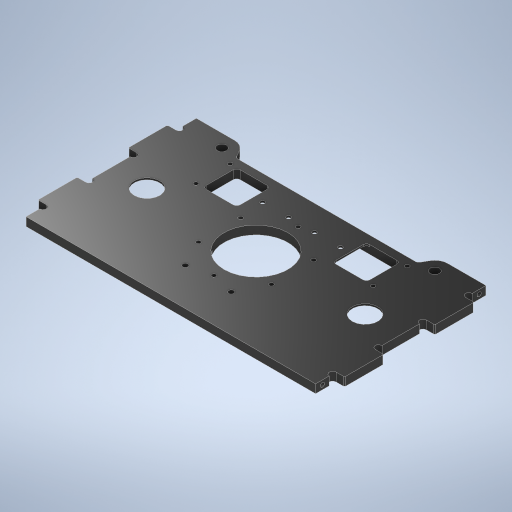
# Autodesk Inventor part: TorsoUpperFrame
Saved by Autodesk Inventor 2024.2 (Build 282272000, 272)
## iProperties
Created: 2024-01-05
Part Number: TorsoUpperFrame
Material: Aluminum 7075
Document SubType Name: Modeling
Designer: Masato Kubotera
Density: 2.81 g/cm^3
Appearance: Glossy - Black
Vendor: meviy
Mass: 108.003 g
Surface Area: 393.241 cm^2
Volume: 38.4352 cm^3
Author: Masato Kubotera
Autodesk Inventor part; units mm, degrees
ref_plane "YZ Plane" through (0, 0, 0) normal (1, 0, 0) x (0, 1, 0)
ref_plane "XZ Plane" through (0, 0, 0) normal (0, 1, 0) x (-1, 0, 0)
ref_plane "XY Plane" through (0, 0, 0) normal (0, 0, 1) x (1, 0, 0)
sketch "Sketch1" plane through (0, 0, 0) normal (0, 0, 1) x (1, 0, 0)
  line L0 (-50, -90) -> (50, -90)
  line L1 (50, -90) -> (50, 90)
  line L2 (50, 90) -> (-50, 90)
  line L3 (-50, 90) -> (-50, -90)
  line L4 (-50, -90) -> (50, 90) construction
  line L5 (50, -90) -> (-50, 90) construction
  line L6 (-50, 0) -> (50, 0)
  line L7 (0, -90) -> (0, 90) construction
  circle A0 centre (0, 0) radius 18.75
  line L8 (-12, -16) -> (31, -16) construction
  line L9 (31, -16) -> (31, 16) construction
  line L10 (31, 16) -> (-12, 16) construction
  line L11 (-12, 16) -> (-12, -16) construction
  line L12 (-12, -16) -> (31, 16) construction
  line L13 (31, -16) -> (-12, 16) construction
  line L14 (1, -13.5) -> (28, -13.5) construction
  line L15 (28, -13.5) -> (28, 13.5) construction
  line L16 (28, 13.5) -> (1, 13.5) construction
  line L17 (1, 13.5) -> (1, -13.5) construction
  line L18 (1, -13.5) -> (28, 13.5) construction
  line L19 (28, -13.5) -> (1, 13.5) construction
  line L20 (9.61, -16.1) -> (31.1, -16.1)
  line L21 (31.1, -16.1) -> (31.1, 16.1)
  line L22 (31.1, 16.1) -> (9.61, 16.1)
  line L23 (50, 85) -> (38, 85)
  line L24 (38, 85) -> (38, 90)
  line L25 (-15, 90) -> (-15, 85)
  line L26 (-15, 85) -> (15, 85)
  line L27 (15, 85) -> (15, 90)
  arc A1 (38, 85) -> (42, 85) centre (40, 85) ccw
  arc A2 (11, 85) -> (15, 85) centre (13, 85) ccw
  line L28 (-50, 85) -> (-38, 85)
  line L29 (-38, 85) -> (-38, 90)
  arc A3 (-42, 85) -> (-38, 85) centre (-40, 85) ccw
  arc A4 (-15, 85) -> (-11, 85) centre (-13, 85) ccw
  line L30 (46, 85) -> (46, 79) construction
  line L31 (-46, 85) -> (-46, 79) construction
  circle A5 centre (0, 0) radius 29 construction
  line L32 (-41.5, 0) -> (-41.5, 53.2624)
  line L33 (-41.5, 53.2624) -> (-50, 58.1699)
  circle A6 centre (-42.5, 62.5) radius 7.5 construction
  circle A7 centre (-42.5, 62.5) radius 5 construction
  line L34 (-70, -90.6743) -> (-70, 90) construction
  line L35 (70, -90.6743) -> (70, 90) construction
  line L36 (-50, 62.5) -> (-37.5, 62.5) construction
  circle A8 centre (-42.5, -62.5) radius 7.5 construction
  circle A9 centre (-42.5, -62.5) radius 5 construction
  line L37 (50, -85) -> (38, -85)
  line L38 (38, -85) -> (38, -90)
  line L39 (-15, -90) -> (-15, -85)
  line L40 (-15, -85) -> (15, -85)
  line L41 (15, -85) -> (15, -90)
  arc A10 (42, -85) -> (38, -85) centre (40, -85) ccw
  arc A11 (15, -85) -> (11, -85) centre (13, -85) ccw
  arc A12 (-11, -85) -> (-15, -85) centre (-13, -85) ccw
  line L42 (-38, -85) -> (-38, -90)
  arc A13 (-38, -85) -> (-42, -85) centre (-40, -85) ccw
  line L43 (-50, -85) -> (-38, -85)
  line L44 (-41.5, 0) -> (-41.5, -53.2624)
  line L45 (-41.5, -53.2624) -> (-50, -58.1699)
  line L46 (-35.6, 29.25) -> (-17.9, 29.25) construction
  line L47 (-17.4, 28.75) -> (-36.1, 28.75) construction
  line L48 (-36.6858, 30.1642) -> (-36.6858, 46.0358)
  line L49 (-35.6, 46.95) -> (-35.6, 29.25) construction
  line L50 (-35.6, 46.95) -> (-17.9, 29.25) construction
  line L51 (-17.9, 46.95) -> (-35.6, 29.25) construction
  line L52 (-36.1, 47.45) -> (-17.4, 47.45) construction
  line L53 (-36.1, 47.45) -> (-17.4, 28.75) construction
  line L54 (-17.4, 47.45) -> (-36.1, 28.75) construction
  line L55 (-36.6858, 48.0358) -> (-16.8142, 28.1642) construction
  line L56 (-16.8142, 48.0358) -> (-36.6858, 28.1642) construction
  arc A14 (-34.6858, 48.0358) -> (-36.6858, 46.0358) centre (-34.6858, 46.0358) ccw
  line L57 (-16.8142, 46.0358) -> (-16.8142, 30.1642)
  line L58 (-17.9, 29.25) -> (-17.9, 46.95) construction
  line L59 (-17.4, 47.45) -> (-17.4, 28.75) construction
  line L60 (-18.8142, 28.1642) -> (-34.6858, 28.1642)
  arc A15 (-36.6858, 30.1642) -> (-34.6858, 28.1642) centre (-34.6858, 30.1642) ccw
  arc A16 (-18.8142, 28.1642) -> (-16.8142, 30.1642) centre (-18.8142, 30.1642) ccw
  line L61 (-34.6858, 48.0358) -> (-18.8142, 48.0358)
  arc A17 (-16.8142, 46.0358) -> (-18.8142, 48.0358) centre (-18.8142, 46.0358) ccw
  line L62 (-17.9, 46.95) -> (-35.6, 46.95) construction
  line L63 (-36.1, 28.75) -> (-36.1, 47.45) construction
  line L64 (-36.6858, -30.1642) -> (-36.6858, -46.0358)
  line L65 (-34.6858, -48.0358) -> (-18.8142, -48.0358)
  line L66 (-35.6, -46.95) -> (-35.6, -29.25) construction
  line L67 (-17.9, -46.95) -> (-35.6, -46.95) construction
  line L68 (-36.1, -28.75) -> (-36.1, -47.45) construction
  line L69 (-36.1, -47.45) -> (-17.4, -47.45) construction
  line L70 (-35.6, -29.25) -> (-17.9, -29.25) construction
  line L71 (-35.6, -46.95) -> (-17.9, -29.25) construction
  line L72 (-17.9, -46.95) -> (-35.6, -29.25) construction
  line L73 (-18.8142, -28.1642) -> (-34.6858, -28.1642)
  line L74 (-16.8142, -48.0358) -> (-36.6858, -28.1642) construction
  line L75 (-36.6858, -48.0358) -> (-16.8142, -28.1642) construction
  line L76 (-17.4, -28.75) -> (-36.1, -28.75) construction
  line L77 (-36.1, -47.45) -> (-17.4, -28.75) construction
  line L78 (-17.4, -47.45) -> (-36.1, -28.75) construction
  line L79 (-17.9, -29.25) -> (-17.9, -46.95) construction
  line L80 (-17.4, -47.45) -> (-17.4, -28.75) construction
  arc A18 (-16.8142, -30.1642) -> (-18.8142, -28.1642) centre (-18.8142, -30.1642) ccw
  line L81 (-16.8142, -46.0358) -> (-16.8142, -30.1642)
  arc A19 (-34.6858, -28.1642) -> (-36.6858, -30.1642) centre (-34.6858, -30.1642) ccw
  arc A20 (-18.8142, -48.0358) -> (-16.8142, -46.0358) centre (-18.8142, -46.0358) ccw
  arc A21 (-36.6858, -46.0358) -> (-34.6858, -48.0358) centre (-34.6858, -46.0358) ccw
  arc A22 (0, 16) -> (-12, 10.583) centre (0, 0) ccw construction
  arc A23 (-12, -10.583) -> (0, -16) centre (0, 0) ccw construction
  line L82 (-26.75, 38.1) -> (-26.75, -38.1) construction
  line L83 (-14.5, 55) -> (-27.6628, 55)
  arc A24 (-39.3295, 80) -> (-41.0778, 77.0287) centre (-39.3295, 78) ccw
  line L84 (-41.5, 16) -> (-37.5, 16) construction
  line L85 (-41.5, -16) -> (-37.5, -16) construction
  line L86 (-37.25, -49) -> (-16.25, -49) construction
  line L87 (-14.25, -47) -> (-14.25, 47) construction
  line L88 (-16.25, 49) -> (-37.25, 49) construction
  line L89 (-39.25, 47) -> (-39.25, -47) construction
  line L90 (-39.25, -49) -> (-14.25, 49) construction
  line L91 (-14.25, -49) -> (-39.25, 49) construction
  line L92 (-16.75, 52) -> (-36.75, 52) construction
  circle A25 centre (-16.75, 52) radius 1 construction
  circle A26 centre (-16.75, 52) radius 2 construction
  line L93 (-39, -55) -> (-14.5, -55) construction
  line L94 (-12.5, -53) -> (-12.5, 53) construction
  line L95 (-14.5, 55) -> (-39, 55) construction
  line L96 (-41, 53) -> (-41, -53) construction
  line L97 (-41, -55) -> (-12.5, 55) construction
  line L98 (-12.5, -55) -> (-41, 55) construction
  arc A27 (-12.5, 53) -> (-14.5, 55) centre (-14.5, 53) ccw
  arc A28 (-39, 55) -> (-41, 53) centre (-39, 53) ccw construction
  arc A29 (-41, -53) -> (-39, -55) centre (-39, -53) ccw construction
  arc A30 (-14.5, -55) -> (-12.5, -53) centre (-14.5, -53) ccw construction
  arc A31 (-37.25, 49) -> (-39.25, 47) centre (-37.25, 47) ccw construction
  arc A32 (-14.25, 47) -> (-16.25, 49) centre (-16.25, 47) ccw construction
  arc A33 (-16.25, -49) -> (-14.25, -47) centre (-16.25, -47) ccw construction
  arc A34 (-39.25, -47) -> (-37.25, -49) centre (-37.25, -47) ccw construction
  line L99 (-17.75, 22.5) -> (-35.75, 22.5) construction
  line L100 (-35.75, 22.5) -> (-35.75, -22.5) construction
  line L101 (-35.75, -22.5) -> (-17.75, -22.5) construction
  line L102 (-17.75, -22.5) -> (-17.75, 22.5) construction
  line L103 (-17.75, 22.5) -> (-35.75, -22.5) construction
  line L104 (-35.75, 22.5) -> (-17.75, -22.5) construction
  line L105 (41.0778, 77.0287) -> (13.0754, 26.6244)
  line L106 (15.6978, 25.1674) -> (43.2517, 74.7643)
  line L107 (47, 73.7931) -> (47, 3.5)
  line L108 (29.1, 18.1) -> (17.9933, 18.1)
  arc A35 (47, 73.7931) -> (43.2517, 74.7643) centre (45, 73.7931) ccw
  arc A36 (16.0474, 20.5621) -> (17.9933, 18.1) centre (17.9933, 20.1) ccw
  line L109 (-36.6858, 23.1642) -> (-36.6858, 0)
  line L110 (-34.37, -22.5) -> (-34.37, 22.5) construction
  line L111 (-29.25, 5.12) -> (-24.25, 5.12) construction
  line L112 (-24.25, 5.12) -> (-24.25, 10.12) construction
  line L113 (-24.25, 10.12) -> (-29.25, 10.12) construction
  line L114 (-29.25, 10.12) -> (-29.25, 5.12) construction
  line L115 (-29.25, 5.12) -> (-24.25, 10.12) construction
  line L116 (-24.25, 5.12) -> (-29.25, 10.12) construction
  circle A37 centre (-26.75, 7.62) radius 1.5 construction
  line L117 (-32.99, -22.5) -> (-32.99, 22.5) construction
  line L118 (-29.25, 25.36) -> (-29.25, 20.36) construction
  line L119 (-29.25, 20.36) -> (-24.25, 20.36) construction
  line L120 (-24.25, 20.36) -> (-24.25, 25.36) construction
  circle A38 centre (-26.75, 22.86) radius 1.5 construction
  line L121 (-24.25, 25.36) -> (-29.25, 25.36) construction
  arc A39 (-23.5471, 4.0762) -> (-29, 0) centre (-24.75, 0) ccw
  arc A40 (-23.5471, 4.0762) -> (-21.0458, 5.4896) centre (-22.9811, 5.9944) ccw
  arc A41 (-17.2299, 13.2738) -> (-21.0458, 5.4896) centre (0, 0) ccw
  arc A42 (5.7687, 20.971) -> (-5.7687, 20.971) centre (0, 0) ccw
  arc A43 (5.7687, 20.971) -> (8.2434, 22.4305) centre (6.2992, 22.8994) ccw
  arc A44 (11.6624, 25.624) -> (13.0754, 26.6244) centre (11.3271, 27.5956) ccw
  arc A45 (15.6978, 25.1674) -> (15.4533, 24.3645) centre (17.4462, 24.1961) ccw
  line L122 (-12.5, 27.3962) -> (-12.5, 53)
  arc A46 (11.6624, 25.624) -> (8.2434, 22.4305) centre (12.375, 21.4341) ccw
  arc A47 (-8.2434, 22.4305) -> (-5.7687, 20.971) centre (-6.2992, 22.8994) ccw
  arc A48 (-8.2434, 22.4305) -> (-11.1, 25.4884) centre (-12.375, 21.4341) ccw
  arc A49 (-12.5, 27.3962) -> (-11.1, 25.4884) centre (-10.5, 27.3962) ccw
  line L123 (-39.3295, 80) -> (39.3295, 80)
  arc A50 (41.0778, 77.0287) -> (39.3295, 80) centre (39.3295, 78) ccw
  line L124 (45, 1.5) -> (35.1, 1.5)
  line L125 (33.1, 3.5) -> (33.1, 14.1)
  arc A51 (45, 1.5) -> (47, 3.5) centre (45, 3.5) ccw
  arc A52 (33.1, 3.5) -> (35.1, 1.5) centre (35.1, 3.5) ccw
  arc A53 (33.1, 14.1) -> (29.1, 18.1) centre (29.1, 14.1) ccw
  line L126 (-41.0778, 77.0287) -> (-29.4111, 56.0287)
  arc A54 (15.6978, 25.1674) -> (15.6898, 23.2395) centre (17.4462, 24.1961) ccw
  arc A55 (16.0474, 20.5621) -> (15.6898, 23.2395) centre (12.375, 21.4341) ccw
  arc A56 (-29.4111, 56.0287) -> (-27.6628, 55) centre (-27.6628, 57) ccw
  line L127 (-36.6858, 23.1642) -> (-36.6858, 30.1642)
  line L128 (-16.8142, 30.1642) -> (-16.8142, 14.4944)
  arc A57 (-17.2299, 13.2738) -> (-16.8142, 14.4944) centre (-18.8142, 14.4944) ccw
  circle A58 centre (0, 64) radius 7.5
  point P0 (9.5, 0)
  point P1 (14.5, 0)
  point P2 (24.75, 0)
  point P3 (-12.375, 21.4341)
  point P4 (-12.375, -21.4341)
  point P5 (12.375, -21.4341)
  point P6 (-37.5, -62.5)
  point P7 (46, -85)
  point P8 (-46, -85)
  point P9 (-50, -58.1699)
  point P10 (-50, -85)
  point P11 (-38, -90)
  point P12 (-11, -85)
  point P13 (38, -90)
  point P14 (50, -85)
  point P15 (-11, 85)
  point P16 (-50, 85)
  point P17 (50, 69.4499)
  point P18 (50, 77.5499)
  point P19 (-46, -79)
  point P20 (-26.75, 38.1)
  point P21 (-26.75, 38.1)
  point P22 (-26.75, -38.1)
  point P23 (-26.75, 38.1)
  point P24 (18.75, 0)
  point P25 (-18.75, 0)
  point P26 (-35, 55)
  point P27 (-28.8396, 55)
  point P28 (-26.75, 0)
  point P29 (-16.75, -52)
  point P30 (-36.75, -52)
  point P31 (43.8396, 82)
  point P32 (42.2091, 72.8876)
  point P33 (47, 72.8875)
  point P34 (47, 1.5)
  point P35 (33.1, 18.1)
  point P36 (-12.5, 51.9999)
  point P37 (40, 83)
  point P38 (-16.8142, 24.516)
  point P39 (-16.8142, 13.7965)
  dimension "d24" = 58
  dimension "d26" = 10
  dimension "d0" = 100
  dimension "d1" = 180
  dimension "d2" = 37.5
  dimension "d3" = 43
  dimension "d4" = 32
  dimension "d5" = 27
  dimension "d6" = 27
  dimension "d7" = 9.5
  dimension "d8" = 8.5
  dimension "d9" = 0.1
  dimension "d10" = 0.1
  dimension "d15" = 360
  dimension "d17" = 49.5
  dimension "d18" = 5
  dimension "d19" = 30
  dimension "d20" = 12
  dimension "d21" = 2
  dimension "d22" = 6
  dimension "d23" = 8
  dimension "d25" = 15
  dimension "d27" = 140
  dimension "d29" = 125
  dimension "d77" = 2
  dimension "d78" = 17.7
  dimension "d79" = 17.7
  dimension "d80" = 0.5
  dimension "d81" = 76.2
  dimension "d100" = 4
  dimension "d101" = 32
  dimension "d128" = 8.5
  dimension "d130" = 29.5
  dimension "d131" = 25
  dimension "d132" = 98
  dimension "d133" = 2
  dimension "d134" = 4
  dimension "d135" = 20
  dimension "d138" = 0.5
  dimension "d139" = 6
  dimension "d140" = 2
  dimension "d141" = 2
  dimension "d149" = 18
  dimension "d150" = 45
  dimension "d151" = 2
  dimension "d153" = 3
  dimension "d157" = 3
  dimension "d173" = 15.24
  dimension "d176" = 5
  dimension "d178" = 3
  dimension "d181" = 15.24
  dimension "d184" = 15.24
  dimension "d191" = 3
  dimension "d205" = 5
  dimension "d212" = 2
  dimension "d213" = 3
  dimension "d215" = 4
  dimension "d216" = 3
  dimension "d218" = 60
  dimension "d223" = 2
  dimension "d225" = 15
  dimension "d226" = 21
  constraints: 258 end point, 101 point on circle, 88 point on line, 80 symmetric about line, 56 centre point, 54 tangent, 35 midpoint, 22 equal radius, 20 horizontal, 20 parallel, 17 coincident, 13 vertical, 11 perpendicular, 3 collinear, 3 horizontal alignment, 1 concentric, 44 other
  measures "d0" distance of L2.end L1.end
  measures "d1" distance of L1.end L0.end
  measures "d2" diameter of A0
  measures "d3" distance of L10.end L9.end
  measures "d4" distance of L9.end L8.end
  measures "d5" distance of L16.end L15.end
  measures "d6" distance of L15.end L14.end
  measures "d7" distance from line of point (9.5, 0) L7
  measures "d8" distance from line of point (9.5, 0) L17
  measures "d9" distance between parallel lines of L22 L10
  measures "d10" distance between parallel lines of L21 L9
  measures "d17" distance of point (24.75, 0) point (-24.75, 0)
  measures "d18" distance between parallel lines of L2 L23
  measures "d19" distance between parallel lines of L27 L25
  measures "d20" distance from line of L1.end L24
  measures "d21" radius of A1
  measures "d22" distance of L30.start L30.end
  measures "d23" distance between parallel lines of L30 L24
  measures "d25" diameter of A6
  measures "d27" distance between parallel lines of L35 L34
  measures "d29" distance of point (-42.5, 62.5) point (-42.5, -62.5)
  measures "d77" radius of A15
  measures "d78" distance of L46.end L49.end
  measures "d79" distance of L49.end L49.start
  measures "d80" distance between parallel lines of L49 L63
  measures "d81" distance of L82.end point (-26.75, 38.1)
  measures "d100" distance of L84.start L84.end
  measures "d101" distance between parallel lines of L85 L84
  measures "d128" distance between parallel lines of L32 L3
  measures "d130" distance between parallel lines of L11 L32
  measures "d131" distance of L91.end L90.end
  measures "d132" distance of L90.end L91.start
  measures "d133" diameter of A25
  measures "d134" diameter of A26
  measures "d135" distance of L92.start L92.end
  measures "d138" distance between parallel lines of L94 L11
  measures "d139" distance between parallel lines of L95 L88
  measures "d140" radius of A27
  measures "d141" radius of A31
  measures "d149" distance of L101.end L100.end
  measures "d150" distance of L100.end L99.end
  measures "d151" distance between parallel lines of L108 L22
  measures "d153" distance between parallel lines of L106 L105
  measures "d157" distance between parallel lines of L1 L107
  measures "d173" diameter of L110 L82
  measures "d176" distance of L113.end L112.end
  measures "d178" diameter of A37
  measures "d181" diameter of A37.centre L6
  measures "d184" distance of L113.end L118.start
  measures "d191" radial gap between concentric circles of A0 A41
  measures "d205" distance of L111.end L112.end
  measures "d212" distance between parallel lines of L21 L125
  measures "d213" diameter of L124 L6
  measures "d215" radius of A53
  measures "d216" distance from line of point (40, 83) L123
  measures "d218" angle of L3 L33
  measures "d223" radius of A40
  measures "d225" diameter of A58
  measures "d226" distance from line of L26 point (0, 64)
extrude "Extrusion1" add sketch "Sketch1" along normal blind 5 contours L3 L28 A3 L29 L2 L25 A4 L26 A2 L27 L24 A1 L23 L1 L6 L21 L22 A0 A39 A40 A41 A57 L128 L57 A17 L61 A14 L48 L127 L109 L32 L33 | L109 L127 A15 L60 A16 L128 A57 A41 A40 A39 L6 | L6 A0 L22 L21 | L83 A56 L126 A24 L123 A50 L105 A44 A46 A43 A42 A47 A48 A49 L122 A27 | L106 A35 L107 A51 L124 A52 L125 A53 L108 A36 A55 A54 A45
extrude "Extrusion2" cut sketch "Sketch1" along normal blind 2 contours L21 L20 A0 L6 | L6 A0 L22 L21
extrude "Extrusion3" cut sketch "Sketch1" along normal blind 4 contours L109 L127 A15 L60 A16 L128 A57 A41 A40 A39 L6 | L83 A56 L126 A24 L123 A50 L105 A44 A46 A43 A42 A47 A48 A49 L122 A27 | L106 A35 L107 A51 L124 A52 L125 A53 L108 A36 A55 A54 A45 | A58
hole "M3" at (12.375, -21.4341, 0) at (24.75, 0, 0) at (12.375, 21.4341, 0) at (-12.375, 21.4341, 0) at (-12.375, -21.4341, 0) at (-24.75, 0, 0) at (-42.5, -62.5, 0) at (-26.75, 7.62, 0) at (-26.75, 22.86, 0) direction (0, 0, 1) diameter 2.459 end through all thread size "M3x0.5" class "6H" standard "ANSI Metric M Profile"
hole "M4" [suppressed]
hole "Phi3.1" at (28, -13.5, 0) at (28, 13.5, 0) direction (0, 0, 1) diameter 3.1 end through all
hole "Phi5.5" at (-42.5, 62.5, 0) at (-42.5, -62.5, 0) direction (0, 0, 1) diameter 5.5 end through all
sketch "Sketch2" plane through (-11, 85, 0) normal (0, 1, 0) x (1, 0, 0)
  line L0 (44, 0) -> (53, 0) projected
  line L1 (57, 0) -> (57, -5) construction
  line L2 (61, -5) -> (53, -5) projected
  line L3 (61, 0) -> (53, 0) projected
  line L4 (-31, -5) -> (-39, -5) projected
  line L5 (-35, -5) -> (-35, 0) construction
  point P0 (11, 0)
  point P1 (57, -2.5)
  point P2 (-35, -2.5)
  point P3 (-35, 0)
  point P4 (57, 0)
  point P5 (57, -2.5)
  point P6 (-35, -2.5)
  constraints: 5 midpoint, 4 end point, 3 coincident, 2 vertical
hole "Side-M3" at (46, 85, 2.5) at (-46, 85, 2.5) direction (0, -1, 0) diameter 2.459 depth 6 thread size "M3x0.5" class "6H" standard "ANSI Metric M Profile"
hole "Phi2.5" at (-16.75, 52, 0) at (-36.75, 52, 0) at (-16.75, -52, 0) at (-36.75, -52, 0) direction (0, 0, 1) diameter 2.459 end through all thread size "M3x0.5" class "6H" standard "ISO Metric profile"
fillet "R2" radius 2 2 edges at (31.1, 16.1, 1) (-41.5, 53.2624, 2.5)
chamfer "C0.5" distance 0.5 angle 45 4 edges at (38, 90, 2.5) (15, 90, 2.5) (-15, 90, 2.5) (-38, 90, 2.5)
mirror "Mirror1" about plane through (0, 0, 0) normal (0, 1, 0)
sketch "Sketch3" plane through (-41.5, 52.1077, 0) normal (-1, 0, 0) x (0, 0, 1)
  line L0 (5, 0) -> (5, -104.2154) projected
  line L1 (5, -36.1077) -> (0, -36.1077)
  line L2 (5, -68.1077) -> (0, -68.1077)
  point P0 (0, -52.1077)
  point P1 (2.5, -36.1077)
  point P2 (0, -68.1077)
  point P3 (2.5, -68.1077)
  constraints: 4 end point, 2 coincident, 2 horizontal, 2 midpoint, 2 point on line
hole "Side-M2" [suppressed]
fillet "Fillet2" radius 7.5 2 edges at (-50, 58.1699, 2.5) (-50, -58.1699, 2.5)
equation "\"d10\" = d9"
body "Solid1"
